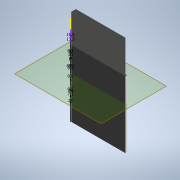
# Autodesk Inventor part: LPS_cap
Saved by Autodesk Inventor 2022 (Build 260153000, 153)
## iProperties
Created: 2024-07-06
Part Number: LPS_cap
Material: Типовые
Document SubType Name: Modeling
Designer: Капустяник Андрей
Density: 1 g/cm^3
Appearance: По умолчанию
Author: Капустяник Андрей
Autodesk Inventor part; units mm, degrees
ref_plane "YZ Plane" through (0, 0, 0) normal (1, 0, 0) x (0, 1, 0)
ref_plane "XZ Plane" through (0, 0, 0) normal (0, 1, 0) x (-1, 0, 0)
sketch "Эскиз1" plane through (0, 0, 0) normal (0, 0, 1) x (1, 0, 0)
  line L0 (-77.0756, -58) -> (-77.0756, 58) projected
  line L1 (-77.0756, 58) -> (67.0756, 58) projected
  line L2 (67.0756, 58) -> (67.0756, -58) projected
  line L3 (67.0756, -58) -> (-77.0756, -58) projected
  line L4 (-77.0756, -58) -> (-77.0756, 58) projected
  line L5 (9.0756, -58) -> (-77.0756, -58) projected
  line L6 (-77.0756, 58) -> (9.0756, 58) projected
  point P0 (0, 0)
extrude "Выдавливание1" add sketch "Эскиз1" along normal blind 3
sketch "Эскиз2" plane through (0, 0, 0) normal (0, 0, -1) x (-1, 0, 0)
  line L0 (-64.0756, 55) -> (74.0756, 55) projected
  line L1 (74.0756, 55) -> (74.0756, -55) projected
  line L2 (74.0756, -55) -> (-64.0756, -55) projected
  line L3 (-64.0756, -55) -> (-64.0756, 55) projected
  line L4 (77.0756, -58) -> (77.0756, 58) projected
  line L5 (77.0756, 58) -> (-67.0756, 58) projected
  line L6 (-67.0756, 58) -> (-67.0756, -58) projected
  line L7 (-67.0756, -58) -> (77.0756, -58) projected
  line L8 (-67.0756, -58) -> (-67.0756, 58) projected
  line L9 (-67.0756, 58) -> (77.0756, 58) projected
  line L10 (77.0756, 58) -> (77.0756, -58) projected
  line L11 (77.0756, -58) -> (-67.0756, -58) projected
  line L12 (-9.0756, 55) -> (74.0756, 55)
  line L13 (74.0756, 55) -> (74.0756, -55)
  line L14 (74.0756, -55) -> (-9.0756, -55)
  point P0 (0, 0)
  point P1 (68.51, 55)
  point P2 (68.51, -55)
  constraints: 6 end point, 2 horizontal, 1 vertical, 4 other
ref_plane "РабПлоскость1" through (-68.51, -58, -55) normal (0, 0, 1) x (1, 0, 0)
extrude "Выдавливание2" add sketch "Эскиз2" along normal up to surface (55 mm away)
chamfer "Фаска1" distance 50 angle 45 1 edges at (-77.0756, 0, 3)
sketch "Эскиз4" plane through (-27.7928, -58, 2.2828) normal (-0.7071068, 0, 0.7071068) x (0.7071068, 0, 0.7071068)
  line L0 (-3.2284, 3) -> (-65.4538, 3) projected
  line L1 (-65.4538, 3) -> (-65.4538, 113) projected
  line L2 (-65.4538, 113) -> (-3.2284, 113) projected
  line L3 (-3.2284, 113) -> (-3.2284, 3) projected
  line L4 (-69.6964, 0) -> (1.0143, 0) projected
  line L5 (1.0143, 0) -> (1.0143, 116) projected
  line L6 (1.0143, 116) -> (-69.6964, 116) projected
  line L7 (-69.6964, 116) -> (-69.6964, 0) projected
  point P0 (18.0383, 58)
extrude "Выдавливание4" add sketch "Эскиз4" against normal blind 3 contours L0 L1 L2 L3 | L7 L6 L5 L4
sketch "Эскиз9" plane through (-28.51, -58, 3) normal (-0.7071068, 0, 0.7071068) x (0.7071068, 0, 0.7071068)
  line L0 (-10, 105.175) -> (-30, 105.175)
  line L1 (-30, 105.175) -> (-30, 91.875)
  line L2 (-30, 91.875) -> (-10, 91.875)
  line L3 (-10, 91.875) -> (-10, 105.175)
  circle A0 centre (-43.2843, 98.525) radius 5.25
  line L4 (-7, 80.55) -> (-33, 80.55)
  line L5 (-33, 80.55) -> (-33, 35.45)
  line L6 (-33, 35.45) -> (-7, 35.45)
  line L7 (-7, 35.45) -> (-7, 80.55)
  line L8 (-33.5, 34.95) -> (-33.5, 81.05)
  line L9 (-33.5, 81.05) -> (-6.5, 81.05)
  line L10 (-6.5, 81.05) -> (-6.5, 34.95)
  line L11 (-6.5, 34.95) -> (-33.5, 34.95)
  line L12 (-6.5, 70.5) -> (-33.5, 70.5)
  line L13 (-33.5, 70.5) -> (-33.5, 45.5)
  line L14 (-33.5, 45.5) -> (-6.5, 45.5)
  line L15 (-6.5, 45.5) -> (-6.5, 70.5)
  line L16 (-6.5, 70.5) -> (-6, 70.5)
  line L17 (-6, 70.5) -> (-6, 45.5)
  line L18 (-6, 45.5) -> (-6.5, 45.5)
  line L19 (-6.5, 45.5) -> (-6.5, 70.5)
  line L20 (-33.5, 70.5) -> (-34, 70.5)
  line L21 (-34, 70.5) -> (-34, 45.5)
  line L22 (-34, 45.5) -> (-33.5, 45.5)
  line L23 (-33.5, 45.5) -> (-33.5, 70.5)
  line L24 (0, 0) -> (0, 116) projected
  line L25 (0, 116) -> (0, 0)
  line L26 (0, 0) -> (0, 58)
  line L27 (0, 58) -> (-56.5685, 58)
  line L28 (-56.5685, 116) -> (-56.5685, 0) projected
  circle A1 centre (-15.7843, 17.475) radius 3.65
  circle A2 centre (-40.7843, 17.475) radius 3.65
  line L29 (-6.5, 34.95) -> (-6.5, 0)
  line L30 (-56.5685, 0) -> (0, 0) projected
  line L31 (-6.5, 17.475) -> (-56.5685, 17.475)
  line L32 (-56.5685, 17.475) -> (0, 17.475)
  line L33 (-15.7843, 17.475) -> (-40.7843, 17.475)
  circle A3 centre (-45.0343, 73.55) radius 4.15
  line L34 (-56.5685, 81.05) -> (-33.5, 81.05)
  line L35 (-33.5, 81.05) -> (-33.5, 34.95)
  line L36 (-33.5, 34.95) -> (-56.5685, 34.95)
  line L37 (-56.5685, 34.95) -> (-56.5685, 81.05)
  line L38 (-45.0343, 81.05) -> (-45.0343, 34.95)
  circle A4 centre (-45.0343, 73.55) radius 7.5
  line L39 (-6.5, 81.05) -> (-6.5, 116)
  line L40 (-6.5, 98.525) -> (-56.5685, 98.525)
  line L41 (-56.5685, 98.525) -> (0, 98.525)
  line L42 (-30, 98.525) -> (-56.5685, 98.525)
  line L43 (-20, 91.875) -> (-20, 0)
  point P0 (18.0383, 58)
  point P1 (-6.5, 58)
  point P2 (-6.5, 58)
  point P3 (-28.2843, 17.475)
  point P4 (-10, 98.525)
  point P5 (-20, 81.05)
  dimension "d31" = 20
  dimension "d32" = 13.3
  dimension "d33" = 10.5
  dimension "d34" = 26
  dimension "d35" = 45.1
  dimension "d36" = 0.5
  dimension "d37" = 25
  dimension "d38" = 0.5
  dimension "d39" = 0.5
  dimension "d40" = 7.3
  dimension "d41" = 7.3
  dimension "d45" = 25
  dimension "d46" = 8.3
  dimension "d47" = 15
  dimension "d48" = 10
  constraints: 82 end point, 20 point on line, 16 midpoint, 15 equal length, 11 perpendicular, 6 horizontal, 5 centre point, 4 collinear, 3 coincident, 2 vertical, 1 tangent, 3 other
  measures "d31" distance of L2.end L1.end
  measures "d32" distance of L1.end L0.end
  measures "d33" diameter of A0
  measures "d34" distance of L6.end L5.end
  measures "d35" distance of L5.end L4.end
  measures "d36" distance between parallel lines of L5 L8
  measures "d37" distance of L13.end L12.end
  measures "d38" distance of L17.end L18.end
  measures "d39" distance of L22.end L21.end
  measures "d40" diameter of A1
  measures "d41" diameter of A2
  measures "d45" distance of L33.start L33.end
  measures "d46" diameter of A3
  measures "d47" diameter of A4
  measures "d48" distance between parallel lines of L25 L3
sketch "Эскиз10" plane through (-28.51, -58, 3) normal (-0.7071068, 0, 0.7071068) x (0.7071068, 0, 0.7071068)
  line L0 (-30, 105.175) -> (-30, 91.875) projected
  line L1 (-10, 105.175) -> (-30, 105.175) projected
  line L2 (-30, 91.875) -> (-10, 91.875) projected
  line L3 (-10, 91.875) -> (-10, 105.175) projected
  circle A0 centre (-43.2843, 98.525) radius 5.25 projected
  circle A1 centre (-45.0343, 73.55) radius 4.15 projected
  circle A2 centre (-40.7843, 17.475) radius 3.65 projected
  circle A3 centre (-15.7843, 17.475) radius 3.65 projected
  line L4 (-6.5, 34.95) -> (-33.5, 34.95) projected
  line L5 (-33.5, 34.95) -> (-33.5, 81.05) projected
  line L6 (-34, 70.5) -> (-34, 45.5) projected
  line L7 (-33.5, 81.05) -> (-6.5, 81.05) projected
  line L8 (-6.5, 81.05) -> (-6.5, 34.95) projected
  line L9 (-6.5, 70.5) -> (-6, 70.5) projected
  line L10 (-6, 70.5) -> (-6, 45.5) projected
  line L11 (-6, 45.5) -> (-6.5, 45.5) projected
  line L12 (-33.5, 70.5) -> (-34, 70.5) projected
  line L13 (-34, 45.5) -> (-33.5, 45.5) projected
  line L14 (-6.15, 69.35) -> (-6.15, 60.2) projected
  point P0 (18.0383, 58)
extrude "Выдавливание9" [suppressed]
sketch "Эскиз11" plane through (-25.6715, -58, 0.1615) normal (0.7071068, 0, -0.7071068) x (-0.7071068, 0, -0.7071068)
  line L0 (0.2284, 3) -> (0.2284, 113) projected
  line L1 (40.7843, 17.475) -> (40.7843, 25.8116)
  line L2 (38.9594, 25.1915) -> (38.9372, 24.9384) projected
  arc A0 (38.8018, 24.8228) -> (38.9372, 24.9384) centre (38.8107, 24.9495) ccw projected
  arc A1 (38.8018, 24.8228) -> (37.7667, 24.8228) centre (38.2843, 17.475) ccw projected
  arc A2 (38.9594, 25.1915) -> (38.8419, 25.3292) centre (38.8329, 25.2026) ccw projected
  arc A3 (37.6313, 24.9384) -> (37.7667, 24.8228) centre (37.7578, 24.9495) ccw projected
  line L3 (37.6092, 25.1915) -> (37.6313, 24.9384) projected
  arc A4 (37.7267, 25.3292) -> (37.6092, 25.1915) centre (37.7357, 25.2026) ccw projected
  arc A5 (39.3003, 25.2832) -> (37.2683, 25.2832) centre (38.2843, 17.475) ccw projected
  arc A6 (40.1771, 26.0275) -> (39.4118, 25.1305) centre (40.2357, 25.2026) ccw
  line L4 (39.4118, 25.1305) -> (39.434, 24.8774)
  arc A7 (39.434, 24.8774) -> (40.3159, 24.1245) centre (40.2578, 24.9495) ccw
  arc A8 (41.2526, 24.1245) -> (40.3159, 24.1245) centre (40.7843, 17.475) ccw
  arc A9 (41.2526, 24.1245) -> (42.1346, 24.8774) centre (41.3107, 24.9495) ccw
  line L5 (42.1346, 24.8774) -> (42.1567, 25.1305)
  arc A10 (42.1567, 25.1305) -> (41.3914, 26.0275) centre (41.3329, 25.2026) ccw
  circle A11 centre (40.7843, 17.475) radius 8.574
  arc A12 (-9.3529, 50.5788) -> (-10.2349, 51.3317) centre (-10.1768, 50.5067) ccw
  arc A13 (-11.1715, 51.3317) -> (-10.2349, 51.3317) centre (-10.7032, 57.9812) ccw
  arc A14 (-11.1715, 51.3317) -> (-12.0535, 50.5788) centre (-11.2297, 50.5067) ccw
  arc A15 (-12.0756, 50.3258) -> (-11.3104, 49.4288) centre (-11.2518, 50.2537) ccw
  arc A16 (-10.0961, 49.4288) -> (-9.3308, 50.3258) centre (-10.1546, 50.2537) ccw
  line L6 (-9.3308, 50.3258) -> (-9.3529, 50.5788)
  line L7 (-12.0535, 50.5788) -> (-12.0756, 50.3258)
  circle A17 centre (15.7843, 17.475) radius 8.574
  arc A18 (14.4118, 9.8195) -> (15.1771, 8.9225) centre (15.2357, 9.7474) ccw
  arc A19 (15.3159, 10.8255) -> (14.434, 10.0726) centre (15.2578, 10.0005) ccw
  line L8 (14.434, 10.0726) -> (14.4118, 9.8195)
  arc A20 (15.3159, 10.8255) -> (16.2526, 10.8255) centre (15.7843, 17.475) ccw
  arc A21 (17.1346, 10.0726) -> (16.2526, 10.8255) centre (16.3107, 10.0005) ccw
  arc A22 (16.3914, 8.9225) -> (17.1567, 9.8195) centre (16.3329, 9.7474) ccw
  line L9 (17.1567, 9.8195) -> (17.1346, 10.0726)
  line L10 (0.2284, 113) -> (68.4538, 113) projected
  line L11 (68.4538, 3) -> (0.2284, 3) projected
  line L12 (68.4538, 113) -> (68.4538, 3) projected
  point P0 (-18.0383, 58)
  point P1 (40.1771, 26.0275)
  point P2 (15.1771, 8.9225)
  point P3 (16.3914, 8.9225)
  point P4 (15.1771, 8.9225)
  point P5 (16.3914, 8.9225)
  point P6 (17.1346, 10.0726)
  constraints: 30 point on circle, 16 centre point, 14 end point, 1 vertical, 3 other
extrude "Выдавливание10" [suppressed]
sketch "Эскиз14" plane through (-65.51, -55, -55) normal (1, 0, 0) x (0, 0, -1)
  line L0 (-55, 0) -> (-55, 110) projected
  line L1 (-24.0346, 70.55) -> (-16.7574, 70.55)
  line L2 (-16.7574, 110) -> (-16.7574, 0) projected
  line L3 (-18.0074, 65.55) -> (-15.5074, 65.55)
  line L4 (-15.5074, 65.55) -> (-15.5074, 75.55)
  line L5 (-15.5074, 75.55) -> (-18.0074, 75.55)
  line L6 (-18.0074, 75.55) -> (-18.0074, 65.55)
  line L7 (-18.0074, 65.55) -> (-15.5074, 75.55) construction
  line L8 (-15.5074, 65.55) -> (-18.0074, 75.55) construction
  line L9 (-55, 110) -> (-6.7574, 110) projected
  line L10 (-6.7574, 0) -> (-55, 0) projected
  line L11 (-6.7574, 110) -> (-6.7574, 0) projected
  point P0 (-55, 55)
  dimension "d63" = 2.5
  dimension "d64" = 10
  constraints: 14 end point, 2 horizontal, 2 midpoint, 2 parallel, 1 perpendicular, 1 point on line
  measures "d63" distance of L5.end L4.end
  measures "d64" distance of L4.end L3.end
extrude "Выдавливание13" [suppressed]
ref_plane "РабПлоскость2" through (-65.51, 15.55, -39.4926) normal (0, -1, 0) x (1, 0, 0)
sketch "Эскиз15" plane through (-77.0756, 58, -55) normal (0, 1, 0) x (1, 0, 0)
  line L0 (86.1512, 0) -> (141.1512, -55) projected
  line L1 (144.1512, -55) -> (141.1512, -55) projected
  line L2 (0, 0) -> (86.1512, 0) projected
  line L3 (50, -58) -> (0, -8) projected
  line L4 (144.1512, -58) -> (50, -58) projected
  line L5 (144.1512, 0) -> (144.1512, -58) projected
  line L6 (0, 0) -> (144.1512, 0) projected
  line L7 (0, 0) -> (0, -8) projected
  point P0 (77.0756, -55)
extrude "Выдавливание14" cut sketch "Эскиз15" against normal up to surface (116 mm away) contours L6 L5 L1 L0
